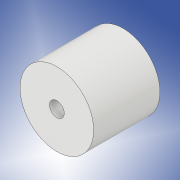
# Autodesk Inventor part: FA012
Saved by Autodesk Inventor 2017 SP1 (Build 210196100, 196)
## iProperties
Created: 2017-07-19
Part Number: FA012
Material: ABS Plastic
Document SubType Name: Modeling
Designer: Zach
Density: 1.06 g/cm^3
Appearance: CR White
Author: Zach
Autodesk Inventor part; units mm, degrees
ref_plane "YZ Plane" through (0, 0, 0) normal (1, 0, 0) x (0, 1, 0)
ref_plane "XZ Plane" through (0, 0, 0) normal (0, 1, 0) x (-1, 0, 0)
ref_plane "XY Plane" through (0, 0, 0) normal (0, 0, 1) x (1, 0, 0)
sketch "Sketch1" plane through (0, 0, 0) normal (0, 0, 1) x (1, 0, 0)
  circle A0 centre (0, 0) radius 15
  dimension "d0" = 30
  constraints: 1 centre point, 1 coincident
  measures "d0" diameter of A0
extrude "Extrusion1" add sketch "Sketch1" along normal blind 19
sketch "Sketch2" plane through (0, 0, 19) normal (0, 0, 1) x (1, 0, 0)
  circle A0 centre (0, 0) radius 3
  dimension "d3" = 6
  constraints: 1 centre point, 1 coincident
  measures "d3" diameter of A0
extrude "Extrusion2" cut sketch "Sketch2" against normal blind 19
sketch "Sketch3" plane through (0, 0, 0) normal (0, 0, -1) x (-1, 0, 0)
  circle A0 centre (0, 0) radius 15 projected
extrude "Extrusion3" add sketch "Sketch3" along normal blind 2
sketch "Sketch4" plane through (0, 0, -2) normal (0, 0, -1) x (-1, 0, 0)
  circle A0 centre (0, 0) radius 3 construction
  line L0 (1.725, 2.9878) -> (3.45, 0)
  line L1 (3.45, 0) -> (1.725, -2.9878)
  line L2 (1.725, -2.9878) -> (-1.725, -2.9878)
  line L3 (-1.725, -2.9878) -> (-3.45, 0)
  line L4 (-3.45, 0) -> (-1.725, 2.9878)
  line L5 (-1.725, 2.9878) -> (1.725, 2.9878)
  point P0 (0, 2.9878)
  dimension "d9" = 6.9
  constraints: 12 end point, 1 coincident, 1 midpoint, 1 vertical alignment, 13 other
  measures "d9" distance of L0.end L3.end
extrude "Extrusion4" add sketch "Sketch4" along normal blind 4
sketch "Sketch5" plane through (0, 0, -2) normal (0, 0, -1) x (-1, 0, 0)
  circle A0 centre (0, 0) radius 3 projected
  circle A1 centre (0, 0) radius 7
  circle A2 centre (0, 0) radius 15 projected
  dimension "d12" = 14
  constraints: 1 centre point, 1 coincident
  measures "d12" diameter of A1
extrude "Extrusion5" add sketch "Sketch5" along normal blind 6 contours A2
body "Solid1"
